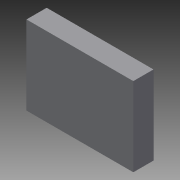
# Autodesk Inventor part: hdd
Saved by Autodesk Inventor 2014 (Build 180170000, 170)
## iProperties
Created: 2015-04-16
Part Number: hdd
Material: Generic
Document SubType Name: Modeling
Designer: Sousaadm
Density: 1 g/cm^3
Appearance: Default
Author: Sousaadm
Autodesk Inventor part; units mm, degrees
ref_plane "YZ Plane" through (0, 0, 0) normal (1, 0, 0) x (0, 1, 0)
ref_plane "XZ Plane" through (0, 0, 0) normal (0, 1, 0) x (-1, 0, 0)
ref_plane "XY Plane" through (0, 0, 0) normal (0, 0, 1) x (1, 0, 0)
sketch "Sketch1" plane through (0, 0, 0) normal (0, 1, 0) x (-1, 0, 0)
  line L0 (-55.5, -41) -> (55.5, -41)
  line L1 (55.5, -41) -> (55.5, 41)
  line L2 (55.5, 41) -> (-55.5, 41)
  line L3 (-55.5, 41) -> (-55.5, -41)
  line L4 (-55.5, -41) -> (55.5, 41) construction
  line L5 (55.5, -41) -> (-55.5, 41) construction
  point P0 (0, 0)
  dimension "d2" = 111
  dimension "d3" = 82
  constraints: 12 end point, 2 midpoint, 2 parallel, 1 horizontal, 1 perpendicular
  measures "d2" distance of L1.end L2.end
  measures "d3" distance of L0.end L1.end
extrude "Extrusion1" add sketch "Sketch1" along normal blind 21
body "Solid1"
